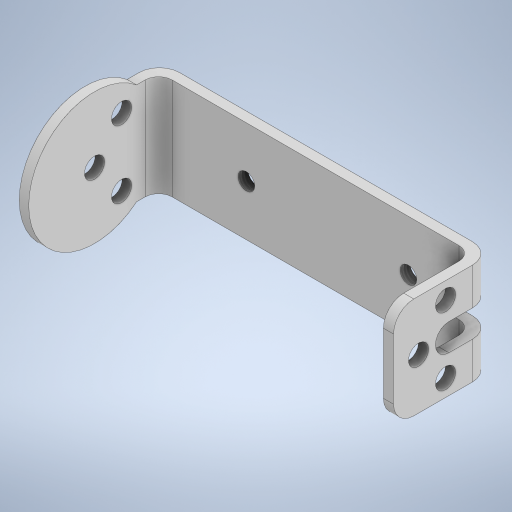
# Autodesk Inventor part: body
Saved by Autodesk Inventor 2024 (Build 280153000, 153)
## iProperties
Created: 2024-09-19
Part Number: body
Material: 一般
Document SubType Name: Modeling
Designer: 1412z
Density: 1 g/cm^3
Appearance: 既定
Author: 1412z
Autodesk Inventor part; units mm, degrees
ref_plane "YZ Plane" through (0, 0, 0) normal (1, 0, 0) x (0, 1, 0)
ref_plane "XZ Plane" through (0, 0, 0) normal (0, 1, 0) x (-1, 0, 0)
ref_plane "XY Plane" through (0, 0, 0) normal (0, 0, 1) x (1, 0, 0)
sketch "スケッチ1" plane through (0, 0, 0) normal (1, 0, 0) x (0, 1, 0)
  circle A0 centre (0, 0) radius 9.75
  dimension "d0" = 19.5
  constraints: 1 centre point, 1 coincident
  measures "d0" diameter of A0
extrude "押し出し1" add sketch "スケッチ1" along normal blind 1.4
sketch "スケッチ2" plane through (1.4, 0, 0) normal (1, 0, 0) x (0, 0, -1)
  circle A0 centre (0, 0) radius 9.75 projected
  line L0 (0, 0) -> (0, -7.5)
  line L1 (0, -7.5) -> (11, -7.5)
  line L2 (11, -7.5) -> (11, 7.5)
  line L3 (11, 7.5) -> (0, 7.5)
  line L4 (0, 7.5) -> (0, 0)
  point P0 (6.23, 7.5)
  point P1 (6.23, -7.5)
  dimension "d3" = 7.5
  dimension "d4" = 11
  dimension "d5" = 15
  constraints: 10 end point, 3 perpendicular, 1 collinear, 1 point on line, 1 vertical
  measures "d3" distance of L0.start L0.end
  measures "d4" distance of L0.end L1.end
  measures "d5" distance of L1.end L2.end
extrude "押し出し2" add sketch "スケッチ2" against normal blind 1.4 contours A0 L3 L2 L1
sketch "スケッチ4" plane through (1.4, 0, 0) normal (1, 0, 0) x (0, 0, -1)
  line L0 (11, -7.5) -> (6.23, -7.5) projected
  line L1 (6.23, 7.5) -> (11, 7.5) projected
  line L2 (11, -7.5) -> (9.5, -7.5)
  line L3 (9.5, -7.5) -> (9.5, 7.5)
  line L4 (9.5, 7.5) -> (11, 7.5)
  line L5 (11, 7.5) -> (11, -7.5)
  point P0 (0, 0)
  dimension "d13" = 1.5
  constraints: 8 end point, 2 parallel, 1 horizontal, 1 perpendicular, 1 point on line
  measures "d13" distance of L3.end L4.end
extrude "押し出し4" add sketch "スケッチ4" along normal blind 48
sketch "スケッチ5" plane through (1.4, -7.5, -9.5) normal (0, 0, 1) x (1, 0, 0)
  line L0 (48, 15) -> (48, 0) projected
  line L1 (48, 15) -> (-1.4, 15) projected
  line L2 (48, 0) -> (46.5, 0)
  line L3 (46.5, 0) -> (46.5, 15)
  line L4 (46.5, 15) -> (48, 15)
  line L5 (48, 15) -> (48, 0)
  point P0 (-1.4, 7.5)
  dimension "d16" = 1.5
  constraints: 8 end point, 2 parallel, 1 horizontal, 1 perpendicular, 1 point on line
  measures "d16" distance of L3.end L4.end
extrude "押し出し5" add sketch "スケッチ5" along normal blind 13.2
sketch "スケッチ6" plane through (0, 0, 0) normal (-1, 0, 0) x (0, 0, 1)
  circle A0 centre (0, 0) radius 1.5
  circle A1 centre (-4, 5) radius 1.5
  circle A2 centre (-4, -5) radius 1.5
  dimension "d19" = 3
  dimension "d20" = 3
  dimension "d21" = 3
  constraints: 3 centre point, 1 coincident
  measures "d19" diameter of A0
  measures "d20" diameter of A1
  measures "d21" diameter of A2
extrude "押し出し6" cut sketch "スケッチ6" against normal blind 50
fillet "フィレット1" radius 3 2 edges at (48.65, 7.5, 3.7) (48.65, -7.5, 3.7)
fillet "フィレット2" radius 3 2 edges at (49.4, 0, -11) (0, 0, -11)
fillet "フィレット3" radius 2 2 edges at (1.4, 0, -9.5) (47.9, 0, -9.5)
sketch "スケッチ7" plane through (46.4, 7.5, -11) normal (0, 0, -1) x (-1, 0, 0)
  circle A0 centre (8, -7.5) radius 1.25
  circle A1 centre (32, -7.5) radius 1.25
  point P0 (46.4, -7.5)
  dimension "d27" = 2.5
  dimension "d28" = 2.5
  constraints: 2 centre point
  measures "d27" diameter of A0
  measures "d28" diameter of A1
extrude "押し出し7" cut sketch "スケッチ7" against normal blind 13.2
sketch "スケッチ8" plane through (49.4, 0, 0) normal (1, 0, 0) x (0, 0, -1)
  line L0 (11, 1.25) -> (11, -1.25) projected
  line L1 (11, 0) -> (11, 2)
  line L2 (11, 7.5) -> (11, -7.5) projected
  line L3 (11, 2) -> (4.5, 2)
  line L4 (4.5, 2) -> (4.5, -2)
  line L5 (4.5, -2) -> (11, -2)
  line L6 (11, -2) -> (11, 0)
  point P0 (0, 0)
  dimension "d31" = 2
  dimension "d32" = 6.5
  dimension "d33" = 4
  constraints: 10 end point, 3 perpendicular, 2 point on line, 1 collinear, 1 midpoint
  measures "d31" distance of L1.start L1.end
  measures "d32" distance of L1.end L3.end
  measures "d33" distance of L3.end L4.end
extrude "押し出し8" cut sketch "スケッチ8" against normal blind 4
sketch "スケッチ9" plane through (49.4, 0, 0) normal (1, 0, 0) x (0, 0, -1)
  line L0 (4.5, 2) -> (4.5, -2) projected
  circle A0 centre (4.5, 0) radius 2
  point P0 (0, 0)
  constraints: 1 midpoint, 3 other
extrude "押し出し9" cut sketch "スケッチ9" against normal blind 4 contours L0 A0 picked at (3.8804, 0.6667)
thread "ねじ1" size "M2.5x0.45" class "6H" standard "ANSI Metric M Profile" full length
thread "ねじ2" size "M2.5x0.45" class "6H" standard "ANSI Metric M Profile" full length
